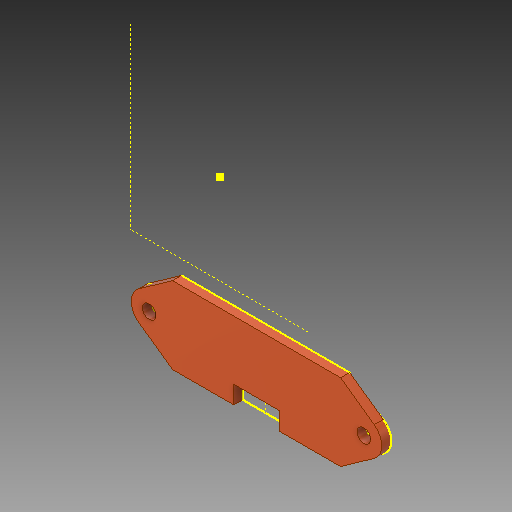
# Autodesk Inventor part: UltrasonicClamp
Saved by Autodesk Inventor 2017 (Build 210142000, 142)
## iProperties
Created: 2017-02-15
Part Number: UltrasonicClamp
Material: Phenolic Resin
Document SubType Name: Modeling
Designer: Moonlight.Admin
Density: 1.38 g/cm^3
Appearance: Smooth - Light Orange
Author: Moonlight.Admin
Autodesk Inventor part; units mm, degrees
ref_plane "YZ Plane" through (0, 0, 0) normal (1, 0, 0) x (0, 1, 0)
ref_plane "XZ Plane" through (0, 0, 0) normal (0, 1, 0) x (-1, 0, 0)
ref_plane "XY Plane" through (0, 0, 0) normal (0, 0, 1) x (1, 0, 0)
derived "CombinedHousingV2.ipt"
sketch "UltrasonicBase" plane through (0, 0, 0) normal (0, 0, 1) x (1, 0, 0)
  line L0 (-10.8, -29.125) -> (36.2, -29.125)
  line L1 (36.2, -29.125) -> (36.2, -50.625)
  line L2 (36.2, -50.625) -> (-10.8, -50.625)
  line L3 (-10.8, -50.625) -> (-10.8, -29.125)
  line L4 (-25.125, -25.125) -> (-25.125, 25.125) construction
  line L5 (25.125, -25.125) -> (-25.125, -25.125) construction
  circle A0 centre (-0.3, -39.875) radius 8.5
  circle A1 centre (25.7, -39.875) radius 8.5
  line L6 (12.7, -50.625) -> (12.7, -29.125) construction
  line L7 (6.35, -50.625) -> (6.35, -45.625)
  line L8 (6.35, -45.625) -> (19.05, -45.625)
  line L9 (19.05, -45.625) -> (19.05, -50.625)
  arc A2 (8.95, -30.125) -> (8.95, -36.125) centre (8.95, -33.125) ccw
  arc A3 (16.45, -36.125) -> (16.45, -30.125) centre (16.45, -33.125) ccw
  line L10 (8.95, -36.125) -> (16.45, -36.125)
  line L11 (8.95, -30.125) -> (16.45, -30.125)
  arc A4 (8.95, -36.125) -> (8.95, -30.125) centre (8.95, -33.125) ccw construction
  arc A5 (16.45, -30.125) -> (16.45, -36.125) centre (16.45, -33.125) ccw construction
  circle A6 centre (-17.3, -39.875) radius 1.905
  circle A7 centre (-17.3, -39.875) radius 5
  circle A8 centre (42.7, -39.875) radius 1.905
  circle A9 centre (42.7, -39.875) radius 5
  point P0 (0, 0)
  point P1 (12.7, -39.875)
sketch "Sketch2" plane through (0, 0, 0) normal (0, 0, 1) x (1, 0, 0)
  circle A0 centre (-17.3, -39.875) radius 1.905 projected
  circle A1 centre (42.7, -39.875) radius 1.905 projected
  circle A2 centre (-17.3, -39.875) radius 5 construction
  circle A3 centre (42.7, -39.875) radius 5 construction
  line L0 (-10.8, -50.625) -> (-10.8, -29.125) construction
  line L1 (36.2, -29.125) -> (36.2, -50.625) construction
  line L2 (-10.8, -29.125) -> (36.2, -29.125)
  line L3 (-10.8, -50.625) -> (6.35, -50.625)
  line L4 (45.5954, -43.9513) -> (36.2, -50.625)
  line L5 (36.2, -29.125) -> (45.5954, -35.7987)
  line L6 (-10.8, -50.625) -> (-20.1954, -43.9513)
  line L7 (-20.1954, -35.7987) -> (-10.8, -29.125)
  arc A4 (45.5954, -43.9513) -> (45.5954, -35.7987) centre (42.7, -39.875) ccw
  arc A5 (-20.1954, -35.7987) -> (-20.1954, -43.9513) centre (-17.3, -39.875) ccw
  line L8 (6.35, -50.625) -> (6.35, -45.625) projected
  line L9 (6.35, -45.625) -> (19.05, -45.625) projected
  line L10 (19.05, -45.625) -> (19.05, -50.625) projected
  line L11 (6.35, -50.625) -> (19.05, -50.625) construction
  line L12 (19.05, -50.625) -> (36.2, -50.625)
  point P0 (0, 0)
  constraints: 18 end point, 8 point on circle, 7 tangent, 3 parallel, 2 centre point, 1 concentric, 1 horizontal
extrude "Extrusion1" add sketch "Sketch2" along normal blind 2.54
body "Solid1"
